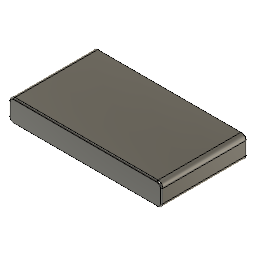
875 8xAA Battery Holder (Autodesk Fusion 360 design; units mm, degrees)
Autodesk Fusion 360 part; units mm, degrees
sketch "Sketch1" plane through (0, 0, 0) normal (0, 0, 1) x (1, 0, 0)
  line L0 (0, 0) -> (127, 0)
  line L1 (127, 0) -> (127, 71)
  line L2 (127, 71) -> (0, 71)
  line L3 (0, 71) -> (0, 0)
  dimension "d1" = 127
  dimension "d2" = 71
  measures "d1" distance of L1.end L2.end
  measures "d2" distance of L0.start L2.end
extrude "Extrude1" add sketch "Sketch1" along normal blind 19
fillet "Fillet1" radius 4 4 edges at (127, 35.5, 19) (127, 35.5, 0) (0, 35.5, 19) (0, 35.5, 0)
fillet "Fillet2" radius 1 16 edges at (63.5, 71, 19) (1.1716, 71, 17.8284) (0, 71, 9.5) (1.1716, 71, 1.1716) (63.5, 71, 0) (125.8284, 71, 1.1716) (127, 71, 9.5) (125.8284, 71, 17.8284) (127, 0, 9.5) (125.8284, 0, 1.1716) (63.5, 0, 0) (1.1716, 0, 1.1716) (0, 0, 9.5) (1.1716, 0, 17.8284) (63.5, 0, 19) (125.8284, 0, 17.8284)
